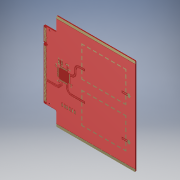
# Autodesk Inventor part: RCS_PCB
Saved by Autodesk Inventor 2018 (Build 220112000, 112)
## iProperties
Created: 2018-01-15
Part Number: RCS_PCB
Material: Epoxy Resin
Document SubType Name: Modeling
Designer: Bradley
Density: 1.14 g/cm^3
Appearance: Red
Author: Bradley
Revision Number: 3
Autodesk Inventor part; units mm, degrees
(part 1 of 4)
ref_plane "YZ Plane" through (0, 0, 0) normal (1, 0, 0) x (0, 1, 0)
ref_plane "XZ Plane" through (0, 0, 0) normal (0, 1, 0) x (-1, 0, 0)
ref_plane "XY Plane" through (0, 0, 0) normal (0, 0, 1) x (1, 0, 0)
sketch "Sketch1" plane through (0, 0, 0) normal (0, 0, 1) x (1, 0, 0)
  line L0 (0, 33.8) -> (12.5, 33.8)
  line L1 (12.5, 33.8) -> (12.5, 47.9)
  line L2 (12.5, 47.9) -> (91.4, 47.9)
  line L3 (91.4, 47.9) -> (91.4, -47.9)
  line L4 (91.4, -47.9) -> (12.5, -47.9)
  line L5 (12.5, -47.9) -> (12.5, -33.8)
  line L6 (12.5, -33.8) -> (0, -33.8)
  line L7 (0, -33.8) -> (0, 33.8)
  line L8 (-4.5, 48) -> (91.5, 48) construction
  line L9 (91.5, 48) -> (91.5, -48) construction
  line L10 (91.5, -48) -> (-4.5, -48) construction
  line L11 (-4.5, -48) -> (-4.5, 48) construction
  line L12 (-4.4, 47.9) -> (-3.4, 47.9) construction
  line L13 (-3.4, 47.9) -> (-3.4, -47.9) construction
  line L14 (-3.4, -47.9) -> (-4.4, -47.9) construction
  line L15 (-4.4, -47.9) -> (-4.4, 47.9) construction
  point P0 (0, 0)
  point P1 (0, 0)
  point P2 (-4.5, 0)
  dimension "d0" = 67.6
  dimension "d1" = 95.8
  dimension "d2" = 91.4
  dimension "d3" = 12.5
  dimension "d20" = 96
  dimension "d21" = 96
  dimension "d22" = 0.1
  dimension "d23" = 0.1
  dimension "d24" = 1
  dimension "d25" = 0.1
  dimension "d26" = 3.4
  constraints: 32 end point, 8 perpendicular, 4 parallel, 3 collinear, 3 horizontal, 2 midpoint, 2 point on line, 1 coincident, 1 horizontal alignment
  measures "d0" distance of L6.end L0.start
  measures "d1" distance of L2.end L3.end
  measures "d2" distance between parallel lines of L7 L3
  measures "d3" distance of L0.start L0.end
  measures "d20" distance of L8.start L8.end
  measures "d21" distance of L10.end L8.start
  measures "d22" distance between parallel lines of L2 L8
  measures "d23" distance between parallel lines of L9 L3
  measures "d24" distance between parallel lines of L15 L13
  measures "d25" distance between parallel lines of L15 L11
  measures "d26" distance between parallel lines of L7 L13
extrude "Extrusion1" add sketch "Sketch1" along normal mid plane 1
sketch "Sketch2" plane through (0, 0, 0.5) normal (0, 0, 1) x (1, 0, 0)
  line L0 (12.5, 33.8) -> (0, 33.8)
  line L1 (0, 33.8) -> (0, -33.8)
  line L2 (0, -33.8) -> (12.5, -33.8)
  line L3 (12.5, -33.8) -> (12.5, -47.9)
  line L4 (12.5, -47.9) -> (91.4, -47.9)
  line L5 (91.4, -47.9) -> (91.4, 47.9)
  line L6 (91.4, 47.9) -> (12.5, 47.9)
  line L7 (12.5, 47.9) -> (12.5, 33.8)
  line L8 (91.4, -47.9) -> (91.4, 47.9)
  line L9 (12.5, 47.9) -> (91.4, 47.9)
  line L10 (91.4, 47.9) -> (91.4, 45.4)
  line L11 (91.4, 45.4) -> (12.5, 45.4)
  line L12 (12.5, 45.4) -> (12.5, 47.9)
  line L13 (91.4, -47.9) -> (12.5, -47.9)
  line L14 (12.5, -47.9) -> (12.5, -45.4)
  line L15 (12.5, -45.4) -> (91.4, -45.4)
  line L16 (91.4, -45.4) -> (91.4, -47.9)
  point P0 (0, 0)
  dimension "d6" = 2.5
  dimension "d27" = 90.8
  constraints: 16 end point, 4 parallel, 2 horizontal, 2 perpendicular, 2 point on line, 1 collinear
  measures "d6" distance between parallel lines of L4 L15
  measures "d27" distance between parallel lines of L15 L11
extrude "Extrusion2" add sketch "Sketch2" along normal blind 0.01 contours L7 L6 L5 L11 | L5 L4 L3 L15
mirror "Mirror1" about plane through (0, 0, 0) normal (0, 0, 1) of "Extrusion2"
sketch "Sketch3" plane through (0, 0, 0.5) normal (0, 0, 1) x (1, 0, 0)
  circle A0 centre (6, 31.8) radius 0.9
  circle A1 centre (6, -31.8) radius 0.9
  point P0 (0, 0)
  dimension "d9" = 1.8
  dimension "d10" = 6
  dimension "d11" = 31.8
  dimension "d12" = 31.8
  constraints: 2 centre point, 1 equal radius, 1 vertical alignment
  measures "d9" diameter of A0
  measures "d10" horizontal distance of point (0, 0) A0.centre
  measures "d11" vertical distance of point (0, 0) A0.centre
  measures "d12" vertical distance of A1.centre point (0, 0)
extrude "Extrusion3" cut sketch "Sketch3" against normal through all
sketch "Sketch4" plane through (0, 0, 0.5) normal (0, 0, 1) x (1, 0, 0)
  circle A0 centre (6, 31.8) radius 0.9
  circle A1 centre (6, -31.8) radius 0.9
  line L0 (12.5, -45.4) -> (91.4, -45.4)
  line L1 (91.4, -45.4) -> (91.4, 45.4)
  line L2 (91.4, 45.4) -> (12.5, 45.4)
  line L3 (12.5, 45.4) -> (12.5, 33.8)
  line L4 (12.5, 33.8) -> (0, 33.8)
  line L5 (0, 33.8) -> (0, -33.8)
  line L6 (0, -33.8) -> (12.5, -33.8)
  line L7 (12.5, -33.8) -> (12.5, -45.4)
  line L8 (0, 18.95) -> (3.5, 18.95)
  arc A2 (3.5, 17.95) -> (3.5, 18.95) centre (3.5, 18.45) ccw
  line L9 (3.5, 17.95) -> (0, 17.95)
  point P0 (0, 0)
  dimension "d15" = 17.95
  dimension "d16" = 3.5
  dimension "d17" = 1
  constraints: 4 end point, 2 point on circle, 2 point on line, 2 tangent, 1 centre point, 1 horizontal, 1 perpendicular
  measures "d15" distance from line of point (0, 0) L9
  measures "d16" distance from line of A2.centre L5
  measures "d17" distance between parallel lines of L9 L8
extrude "Extrusion4" cut sketch "Sketch4" against normal through all contours L5 L8 A2 L9
sketch "Sketch5" plane through (0, 0, 0.5) normal (0, 0, 1) x (1, 0, 0)
  line L0 (37.6, 36.65) -> (82.4, 36.65)
  line L1 (82.4, 36.65) -> (82.4, 5.35)
  line L2 (82.4, 5.35) -> (37.6, 5.35)
  line L3 (37.6, 5.35) -> (37.6, 36.65)
  line L4 (81.4, 35.65) -> (38.6, 35.65)
  line L5 (38.6, 35.65) -> (38.6, 6.35)
  line L6 (38.6, 6.35) -> (81.4, 6.35)
  line L7 (81.4, 6.35) -> (81.4, 35.65)
  line L8 (37.6, 7.9) -> (38.6, 7.9)
  line L9 (37.6, 10.1) -> (38.6, 10.1)
  line L10 (37.6, 13.9) -> (38.6, 13.9)
  line L11 (37.6, 16.1) -> (38.6, 16.1)
  line L12 (37.6, 19.9) -> (38.6, 19.9)
  line L13 (37.6, 22.1) -> (38.6, 22.1)
  line L14 (37.6, 25.9) -> (38.6, 25.9)
  line L15 (37.6, 28.1) -> (38.6, 28.1)
  line L16 (37.6, 31.9) -> (38.6, 31.9)
  line L17 (37.6, 34.1) -> (38.6, 34.1)
  line L18 (81.4, 34.1) -> (82.4, 34.1)
  line L19 (81.4, 31.9) -> (82.4, 31.9)
  line L20 (81.4, 28.1) -> (82.4, 28.1)
  line L21 (81.4, 25.9) -> (82.4, 25.9)
  line L22 (81.4, 22.1) -> (82.4, 22.1)
  line L23 (81.4, 19.9) -> (82.4, 19.9)
  line L24 (81.4, 16.1) -> (82.4, 16.1)
  line L25 (81.4, 13.9) -> (82.4, 13.9)
  line L26 (81.4, 10.1) -> (82.4, 10.1)
  line L27 (81.4, 7.9) -> (82.4, 7.9)
  line L28 (40.9, 6.35) -> (40.9, 5.35)
  line L29 (43.1, 6.35) -> (43.1, 5.35)
  line L30 (46.9, 6.35) -> (46.9, 5.35)
  line L31 (49.1, 6.35) -> (49.1, 5.35)
  line L32 (52.9, 6.35) -> (52.9, 5.35)
  line L33 (55.1, 6.35) -> (55.1, 5.35)
  line L34 (58.9, 6.35) -> (58.9, 5.35)
  line L35 (61.1, 6.35) -> (61.1, 5.35)
  line L36 (64.9, 6.35) -> (64.9, 5.35)
  line L37 (67.1, 6.35) -> (67.1, 5.35)
  line L38 (67.1, 36.65) -> (67.1, 35.65)
  line L39 (64.9, 36.65) -> (64.9, 35.65)
  line L40 (61.1, 36.65) -> (61.1, 35.65)
  line L41 (58.9, 36.65) -> (58.9, 35.65)
  line L42 (55.1, 36.65) -> (55.1, 35.65)
  line L43 (52.9, 36.65) -> (52.9, 35.65)
  line L44 (49.1, 36.65) -> (49.1, 35.65)
  line L45 (46.9, 36.65) -> (46.9, 35.65)
  line L46 (43.1, 36.65) -> (43.1, 35.65)
  line L47 (40.9, 35.65) -> (40.9, 36.65)
  line L48 (83.9, 13.25) -> (86.1, 13.25)
  line L49 (86.1, 13.25) -> (86.1, 16.75)
  line L50 (86.1, 16.75) -> (83.9, 16.75)
  line L51 (83.9, 16.75) -> (83.9, 13.25)
  line L52 (83.9, 14.6) -> (83.4, 14.6)
  line L53 (83.4, 14.6) -> (83.4, 15.4)
  line L54 (83.4, 15.4) -> (83.9, 15.4)
  line L55 (83.9, 15.4) -> (83.9, 14.6)
  line L56 (86.1, 14.6) -> (86.6, 14.6)
  line L57 (86.6, 14.6) -> (86.6, 15.4)
  line L58 (86.6, 15.4) -> (86.1, 15.4)
  line L59 (86.1, 15.4) -> (86.1, 14.6)
  line L60 (70.9, 6.35) -> (70.9, 5.35)
  line L61 (73.1, 6.35) -> (73.1, 5.35)
  line L62 (76.9, 6.35) -> (76.9, 5.35)
  line L63 (79.1, 6.35) -> (79.1, 5.35)
  line L64 (79.1, 35.65) -> (79.1, 36.65)
  line L65 (76.9, 36.65) -> (76.9, 35.65)
  line L66 (73.1, 35.65) -> (73.1, 36.65)
  line L67 (70.9, 36.65) -> (70.9, 35.65)
  point P0 (0, 0)
  point P1 (38.6, 21)
  point P2 (60, 35.65)
  point P3 (83.9, 15)
  point P4 (85, 16.75)
  dimension "d30" = 1
  dimension "d28" = 31.3
  dimension "d29" = 44.8
  dimension "d31" = 60
  dimension "d32" = 21
  dimension "d33" = 2.55
  dimension "d34" = 4.75
  dimension "d35" = 8.55
  dimension "d36" = 10.75
  dimension "d37" = 14.55
  dimension "d38" = 16.75
  dimension "d39" = 20.55
  dimension "d40" = 22.75
  dimension "d41" = 26.55
  dimension "d42" = 28.75
  dimension "d43" = 3.3
  dimension "d44" = 5.5
  dimension "d45" = 9.3
  dimension "d46" = 11.5
  dimension "d47" = 15.3
  dimension "d48" = 17.5
  dimension "d49" = 21.3
  dimension "d50" = 23.5
  dimension "d51" = 27.3
  dimension "d52" = 29.5
  dimension "d55" = 2.2
  dimension "d56" = 3.5
  dimension "d57" = 0.5
  dimension "d58" = 0.8
  dimension "d59" = 15
  dimension "d60" = 85
  dimension "d64" = 33.3
  dimension "d65" = 35.5
  dimension "d66" = 39.3
  dimension "d67" = 41.5
  constraints: 120 end point, 42 point on line, 17 horizontal, 14 vertical, 7 collinear, 6 parallel, 3 midpoint, 3 perpendicular, 122 other
  measures "d28" distance of point (37.6, 5.35) point (37.6, 36.65)
  measures "d29" distance of point (82.4, 5.35) point (37.6, 5.35)
  measures "d31" horizontal distance of point (0, 0) point (60, 35.65)
  measures "d32" vertical distance of point (0, 0) point (38.6, 21)
  measures "d55" distance of L49.end L50.end
  measures "d56" distance of L48.end L49.end
  measures "d57" distance of L53.end L54.end
  measures "d58" distance of L52.end L53.end
  measures "d59" vertical distance of point (83.9, 15) point (0, 0)
  measures "d60" horizontal distance of point (0, 0) point (85, 16.75)
extrude "Extrusion5" add sketch "Sketch5" along normal blind 0.035 contours L0 L47 L4 L5 L17 L3 | L0 L45 L4 L46 | L16 L5 L15 L3 | L0 L43 L4 L44 | L14 L5 L13 L3 | L0 L41 L4 L42 | L12 L5 L11 L3 | L0 L39 L4 L40 | L10 L5 L9 L3 | L0 L67 L4 L38 | L8 L5 L6 L28 L2 L3 | L0 L65 L4 L66 | L29 L6 L30 L2 | L0 L1 L18 L7 L4 L64 | L31 L6 L32 L2 | L1 L20 L7 L19 | L33 L6 L34 L2 | L1 L22 L7 L21 | L35 L6 L36 L2 | L1 L24 L7 L23 | L37 L6 L60 L2 | L1 L26 L7 L25 | L61 L6 L62 L2 | L1 L2 L63 L6 L7 L27 | L51 L50 L49 L48 | L52 L53 L54 L51 | L49 L58 L57 L56
pattern_linear "Rectangular Pattern1" count 2 spacing 40 along (0, -1, 0) of "Extrusion5"
sketch "Sketch6" plane through (0, 0, 0.5) normal (0, 0, 1) x (1, 0, 0)
  line L0 (79.1, -4.35) -> (79.1, -3.35)
  line L1 (79.1, -3.35) -> (82.4, -3.35)
  line L2 (82.4, -3.35) -> (82.4, -5.9)
  line L3 (82.4, -5.9) -> (81.4, -5.9)
  line L4 (81.4, -5.9) -> (81.4, -4.35)
  line L5 (81.4, -4.35) -> (79.1, -4.35)
  line L6 (37.6, -34.65) -> (37.6, -32.1)
  line L7 (37.6, -32.1) -> (38.6, -32.1)
  line L8 (38.6, -32.1) -> (38.6, -33.65)
  line L9 (38.6, -33.65) -> (40.9, -33.65)
  line L10 (40.9, -33.65) -> (40.9, -34.65)
  line L11 (40.9, -34.65) -> (37.6, -34.65)
  line L12 (70.9, -3.35) -> (70.9, -4.35)
  line L13 (70.9, -4.35) -> (67.1, -4.35)
  line L14 (67.1, -4.35) -> (67.1, -3.35)
  line L15 (67.1, -3.35) -> (70.9, -3.35)
  line L16 (73.1, -33.65) -> (76.9, -33.65)
  line L17 (76.9, -33.65) -> (76.9, -34.65)
  line L18 (76.9, -34.65) -> (73.1, -34.65)
  line L19 (73.1, -34.65) -> (73.1, -33.65)
  line L20 (81.4, -20.1) -> (82.4, -20.1)
  line L21 (82.4, -20.1) -> (82.4, -23.9)
  line L22 (82.4, -23.9) -> (81.4, -23.9)
  line L23 (81.4, -23.9) -> (81.4, -20.1)
  line L24 (46.9, -3.35) -> (46.9, -4.35)
  line L25 (46.9, -4.35) -> (43.1, -4.35)
  line L26 (43.1, -4.35) -> (43.1, -3.35)
  line L27 (43.1, -3.35) -> (46.9, -3.35)
  line L28 (58.9, -3.35) -> (58.9, -4.35)
  line L29 (58.9, -4.35) -> (55.1, -4.35)
  line L30 (55.1, -4.35) -> (55.1, -3.35)
  line L31 (55.1, -3.35) -> (58.9, -3.35)
  line L32 (61.1, -33.65) -> (64.9, -33.65)
  line L33 (64.9, -33.65) -> (64.9, -34.65)
  line L34 (64.9, -34.65) -> (61.1, -34.65)
  line L35 (61.1, -34.65) -> (61.1, -33.65)
  line L36 (49.1, -33.65) -> (52.9, -33.65)
  line L37 (52.9, -33.65) -> (52.9, -34.65)
  line L38 (52.9, -34.65) -> (49.1, -34.65)
  line L39 (49.1, -34.65) -> (49.1, -33.65)
  line L40 (81.4, -26.1) -> (82.4, -26.1)
  line L41 (82.4, -26.1) -> (82.4, -29.9)
  line L42 (82.4, -29.9) -> (81.4, -29.9)
  line L43 (81.4, -29.9) -> (81.4, -26.1)
  line L44 (81.4, -8.1) -> (82.4, -8.1)
  line L45 (82.4, -8.1) -> (82.4, -11.9)
  line L46 (82.4, -11.9) -> (81.4, -11.9)
  line L47 (81.4, -11.9) -> (81.4, -8.1)
  line L48 (37.6, -17.9) -> (37.6, -14.1)
  line L49 (37.6, -14.1) -> (38.6, -14.1)
  line L50 (38.6, -14.1) -> (38.6, -17.9)
  line L51 (38.6, -17.9) -> (37.6, -17.9)
  line L52 (86.1, -25.4) -> (86.1, -26.75)
  line L53 (86.1, -26.75) -> (83.9, -26.75)
  line L54 (83.9, -26.75) -> (83.9, -25.4)
  line L55 (83.9, -25.4) -> (83.4, -25.4)
  line L56 (83.4, -25.4) -> (83.4, -24.6)
  line L57 (83.4, -24.6) -> (83.9, -24.6)
  line L58 (83.9, -24.6) -> (83.9, -23.25)
  line L59 (83.9, -23.25) -> (86.1, -23.25)
  line L60 (86.1, -23.25) -> (86.1, -24.6)
  line L61 (86.1, -24.6) -> (86.6, -24.6)
  line L62 (86.6, -24.6) -> (86.6, -25.4)
  line L63 (86.6, -25.4) -> (86.1, -25.4)
  line L64 (37.6, -29.9) -> (37.6, -26.1)
  line L65 (37.6, -26.1) -> (38.6, -26.1)
  line L66 (38.6, -26.1) -> (38.6, -29.9)
  line L67 (38.6, -29.9) -> (37.6, -29.9)
  line L68 (37.6, -11.9) -> (37.6, -8.1)
  line L69 (37.6, -8.1) -> (38.6, -8.1)
  line L70 (38.6, -8.1) -> (38.6, -11.9)
  line L71 (38.6, -11.9) -> (37.6, -11.9)
  line L72 (81.4, -14.1) -> (82.4, -14.1)
  line L73 (82.4, -14.1) -> (82.4, -17.9)
  line L74 (82.4, -17.9) -> (81.4, -17.9)
  line L75 (81.4, -17.9) -> (81.4, -14.1)
  line L76 (43.1, -33.65) -> (46.9, -33.65)
  line L77 (46.9, -33.65) -> (46.9, -34.65)
  line L78 (46.9, -34.65) -> (43.1, -34.65)
  line L79 (43.1, -34.65) -> (43.1, -33.65)
  line L80 (55.1, -33.65) -> (58.9, -33.65)
  line L81 (58.9, -33.65) -> (58.9, -34.65)
  line L82 (58.9, -34.65) -> (55.1, -34.65)
  line L83 (55.1, -34.65) -> (55.1, -33.65)
  line L84 (64.9, -3.35) -> (64.9, -4.35)
  line L85 (64.9, -4.35) -> (61.1, -4.35)
  line L86 (61.1, -4.35) -> (61.1, -3.35)
  line L87 (61.1, -3.35) -> (64.9, -3.35)
  line L88 (52.9, -3.35) -> (52.9, -4.35)
  line L89 (52.9, -4.35) -> (49.1, -4.35)
  line L90 (49.1, -4.35) -> (49.1, -3.35)
  line L91 (49.1, -3.35) -> (52.9, -3.35)
  line L92 (37.6, -23.9) -> (37.6, -20.1)
  line L93 (37.6, -20.1) -> (38.6, -20.1)
  line L94 (38.6, -20.1) -> (38.6, -23.9)
  line L95 (38.6, -23.9) -> (37.6, -23.9)
  line L96 (70.9, -33.65) -> (70.9, -34.65)
  line L97 (70.9, -34.65) -> (67.1, -34.65)
  line L98 (67.1, -34.65) -> (67.1, -33.65)
  line L99 (67.1, -33.65) -> (70.9, -33.65)
  line L100 (76.9, -3.35) -> (76.9, -4.35)
  line L101 (76.9, -4.35) -> (73.1, -4.35)
  line L102 (73.1, -4.35) -> (73.1, -3.35)
  line L103 (73.1, -3.35) -> (76.9, -3.35)
  line L104 (37.6, -3.35) -> (40.9, -3.35)
  line L105 (40.9, -3.35) -> (40.9, -4.35)
  line L106 (40.9, -4.35) -> (38.6, -4.35)
  line L107 (38.6, -4.35) -> (38.6, -5.9)
  line L108 (38.6, -5.9) -> (37.6, -5.9)
  line L109 (37.6, -5.9) -> (37.6, -3.35)
  line L110 (79.1, -33.65) -> (81.4, -33.65)
  line L111 (81.4, -33.65) -> (81.4, -32.1)
  line L112 (81.4, -32.1) -> (82.4, -32.1)
  line L113 (82.4, -32.1) -> (82.4, -34.65)
  line L114 (82.4, -34.65) -> (79.1, -34.65)
  line L115 (79.1, -34.65) -> (79.1, -33.65)
  line L116 (79.1, 35.65) -> (79.1, 36.65)
  line L117 (79.1, 36.65) -> (82.4, 36.65)
  line L118 (82.4, 36.65) -> (82.4, 34.1)
  line L119 (82.4, 34.1) -> (81.4, 34.1)
  line L120 (81.4, 34.1) -> (81.4, 35.65)
  line L121 (81.4, 35.65) -> (79.1, 35.65)
  line L122 (37.6, 5.35) -> (37.6, 7.9)
  line L123 (37.6, 7.9) -> (38.6, 7.9)
  line L124 (38.6, 7.9) -> (38.6, 6.35)
  line L125 (38.6, 6.35) -> (40.9, 6.35)
  line L126 (40.9, 6.35) -> (40.9, 5.35)
  line L127 (40.9, 5.35) -> (37.6, 5.35)
  line L128 (70.9, 36.65) -> (70.9, 35.65)
  line L129 (70.9, 35.65) -> (67.1, 35.65)
  line L130 (67.1, 35.65) -> (67.1, 36.65)
  line L131 (67.1, 36.65) -> (70.9, 36.65)
  line L132 (73.1, 6.35) -> (76.9, 6.35)
  line L133 (76.9, 6.35) -> (76.9, 5.35)
  line L134 (76.9, 5.35) -> (73.1, 5.35)
  line L135 (73.1, 5.35) -> (73.1, 6.35)
  line L136 (81.4, 19.9) -> (82.4, 19.9)
  line L137 (82.4, 19.9) -> (82.4, 16.1)
  line L138 (82.4, 16.1) -> (81.4, 16.1)
  line L139 (81.4, 16.1) -> (81.4, 19.9)
  line L140 (46.9, 36.65) -> (46.9, 35.65)
  line L141 (46.9, 35.65) -> (43.1, 35.65)
  line L142 (43.1, 35.65) -> (43.1, 36.65)
  line L143 (43.1, 36.65) -> (46.9, 36.65)
  line L144 (58.9, 36.65) -> (58.9, 35.65)
  line L145 (58.9, 35.65) -> (55.1, 35.65)
  line L146 (55.1, 35.65) -> (55.1, 36.65)
  line L147 (55.1, 36.65) -> (58.9, 36.65)
  line L148 (61.1, 6.35) -> (64.9, 6.35)
  line L149 (64.9, 6.35) -> (64.9, 5.35)
  line L150 (64.9, 5.35) -> (61.1, 5.35)
  line L151 (61.1, 5.35) -> (61.1, 6.35)
  line L152 (49.1, 6.35) -> (52.9, 6.35)
  line L153 (52.9, 6.35) -> (52.9, 5.35)
  line L154 (52.9, 5.35) -> (49.1, 5.35)
  line L155 (49.1, 5.35) -> (49.1, 6.35)
  line L156 (81.4, 13.9) -> (82.4, 13.9)
  line L157 (82.4, 13.9) -> (82.4, 10.1)
  line L158 (82.4, 10.1) -> (81.4, 10.1)
  line L159 (81.4, 10.1) -> (81.4, 13.9)
  line L160 (81.4, 31.9) -> (82.4, 31.9)
  line L161 (82.4, 31.9) -> (82.4, 28.1)
  line L162 (82.4, 28.1) -> (81.4, 28.1)
  line L163 (81.4, 28.1) -> (81.4, 31.9)
  line L164 (37.6, 22.1) -> (37.6, 25.9)
  line L165 (37.6, 25.9) -> (38.6, 25.9)
  line L166 (38.6, 25.9) -> (38.6, 22.1)
  line L167 (38.6, 22.1) -> (37.6, 22.1)
  line L168 (86.1, 14.6) -> (86.1, 13.25)
  line L169 (86.1, 13.25) -> (83.9, 13.25)
  line L170 (83.9, 13.25) -> (83.9, 14.6)
  line L171 (83.9, 14.6) -> (83.4, 14.6)
  line L172 (83.4, 14.6) -> (83.4, 15.4)
  line L173 (83.4, 15.4) -> (83.9, 15.4)
  line L174 (83.9, 15.4) -> (83.9, 16.75)
  line L175 (83.9, 16.75) -> (86.1, 16.75)
  line L176 (86.1, 16.75) -> (86.1, 15.4)
  line L177 (86.1, 15.4) -> (86.6, 15.4)
  line L178 (86.6, 15.4) -> (86.6, 14.6)
  line L179 (86.6, 14.6) -> (86.1, 14.6)
  line L180 (37.6, 10.1) -> (37.6, 13.9)
  line L181 (37.6, 13.9) -> (38.6, 13.9)
  line L182 (38.6, 13.9) -> (38.6, 10.1)
  line L183 (38.6, 10.1) -> (37.6, 10.1)
  line L184 (37.6, 28.1) -> (37.6, 31.9)
  line L185 (37.6, 31.9) -> (38.6, 31.9)
  line L186 (38.6, 31.9) -> (38.6, 28.1)
  line L187 (38.6, 28.1) -> (37.6, 28.1)
  line L188 (81.4, 25.9) -> (82.4, 25.9)
  line L189 (82.4, 25.9) -> (82.4, 22.1)
  line L190 (82.4, 22.1) -> (81.4, 22.1)
  line L191 (81.4, 22.1) -> (81.4, 25.9)
  line L192 (43.1, 6.35) -> (46.9, 6.35)
  line L193 (46.9, 6.35) -> (46.9, 5.35)
  line L194 (46.9, 5.35) -> (43.1, 5.35)
  line L195 (43.1, 5.35) -> (43.1, 6.35)
  line L196 (55.1, 6.35) -> (58.9, 6.35)
  line L197 (58.9, 6.35) -> (58.9, 5.35)
  line L198 (58.9, 5.35) -> (55.1, 5.35)
  line L199 (55.1, 5.35) -> (55.1, 6.35)
  line L200 (64.9, 36.65) -> (64.9, 35.65)
  line L201 (64.9, 35.65) -> (61.1, 35.65)
  line L202 (61.1, 35.65) -> (61.1, 36.65)
  line L203 (61.1, 36.65) -> (64.9, 36.65)
  line L204 (52.9, 36.65) -> (52.9, 35.65)
  line L205 (52.9, 35.65) -> (49.1, 35.65)
  line L206 (49.1, 35.65) -> (49.1, 36.65)
  line L207 (49.1, 36.65) -> (52.9, 36.65)
  line L208 (37.6, 16.1) -> (37.6, 19.9)
  line L209 (37.6, 19.9) -> (38.6, 19.9)
  line L210 (38.6, 19.9) -> (38.6, 16.1)
  line L211 (38.6, 16.1) -> (37.6, 16.1)
  line L212 (70.9, 6.35) -> (70.9, 5.35)
  line L213 (70.9, 5.35) -> (67.1, 5.35)
  line L214 (67.1, 5.35) -> (67.1, 6.35)
  line L215 (67.1, 6.35) -> (70.9, 6.35)
  line L216 (76.9, 36.65) -> (76.9, 35.65)
  line L217 (76.9, 35.65) -> (73.1, 35.65)
  line L218 (73.1, 35.65) -> (73.1, 36.65)
  line L219 (73.1, 36.65) -> (76.9, 36.65)
  line L220 (37.6, 36.65) -> (40.9, 36.65)
  line L221 (40.9, 36.65) -> (40.9, 35.65)
  line L222 (40.9, 35.65) -> (38.6, 35.65)
  line L223 (38.6, 35.65) -> (38.6, 34.1)
  line L224 (38.6, 34.1) -> (37.6, 34.1)
  line L225 (37.6, 34.1) -> (37.6, 36.65)
  line L226 (79.1, 6.35) -> (81.4, 6.35)
  line L227 (81.4, 6.35) -> (81.4, 7.9)
  line L228 (81.4, 7.9) -> (82.4, 7.9)
  line L229 (82.4, 7.9) -> (82.4, 5.35)
  line L230 (82.4, 5.35) -> (79.1, 5.35)
  line L231 (79.1, 5.35) -> (79.1, 6.35)
  line L232 (0, 18.95) -> (3.5, 18.95)
  arc A0 (3.5, 17.95) -> (3.5, 18.95) centre (3.5, 18.45) ccw
  line L233 (3.5, 17.95) -> (0, 17.95)
  line L234 (0, 17.95) -> (0, -33.8)
  line L235 (0, -33.8) -> (12.5, -33.8)
  line L236 (12.5, -33.8) -> (12.5, -45.4)
  line L237 (12.5, -45.4) -> (91.4, -45.4)
  line L238 (91.4, -45.4) -> (91.4, 45.4)
  line L239 (91.4, 45.4) -> (12.5, 45.4)
  line L240 (12.5, 45.4) -> (12.5, 33.8)
  line L241 (12.5, 33.8) -> (0, 33.8)
  line L242 (0, 33.8) -> (0, 18.95)
  circle A1 centre (6, -31.8) radius 0.9
  circle A2 centre (6, 31.8) radius 0.9
  line L243 (18, -25) -> (19, -25)
  line L244 (19, -25) -> (19, -27.5)
  line L245 (19, -27.5) -> (18, -27.5)
  line L246 (18, -27.5) -> (18, -25)
  line L247 (21.54, -27.5) -> (20.54, -27.5)
  line L248 (21.54, -25) -> (21.54, -27.5)
  line L249 (20.54, -25) -> (21.54, -25)
  line L250 (20.54, -27.5) -> (20.54, -25)
  line L251 (24.08, -27.5) -> (23.08, -27.5)
  line L252 (24.08, -25) -> (24.08, -27.5)
  line L253 (23.08, -25) -> (24.08, -25)
  line L254 (23.08, -27.5) -> (23.08, -25)
  line L255 (26.62, -27.5) -> (25.62, -27.5)
  line L256 (26.62, -25) -> (26.62, -27.5)
  line L257 (25.62, -25) -> (26.62, -25)
  line L258 (25.62, -27.5) -> (25.62, -25)
  line L259 (29.16, -27.5) -> (28.16, -27.5)
  line L260 (29.16, -25) -> (29.16, -27.5)
  line L261 (28.16, -25) -> (29.16, -25)
  line L262 (28.16, -27.5) -> (28.16, -25)
  line L263 (31.7, -27.5) -> (30.7, -27.5)
  line L264 (31.7, -25) -> (31.7, -27.5)
  line L265 (30.7, -25) -> (31.7, -25)
  line L266 (30.7, -27.5) -> (30.7, -25)
  line L267 (16.1, 6.35) -> (16.4, 6.35)
  line L268 (16.4, 6.35) -> (16.4, 5.15)
  line L269 (16.4, 5.15) -> (16.1, 5.15)
  line L270 (16.1, 5.15) -> (16.1, 6.35)
  line L271 (16.1, -5.15) -> (16.4, -5.15)
  line L272 (16.4, -5.15) -> (16.4, -6.35)
  line L273 (16.4, -6.35) -> (16.1, -6.35)
  line L274 (16.1, -6.35) -> (16.1, -5.15)
  line L275 (16.6, 6.35) -> (16.9, 6.35)
  line L276 (16.6, 5.15) -> (16.6, 6.35)
  line L277 (16.9, 6.35) -> (16.9, 5.15)
  line L278 (16.6, -5.15) -> (16.9, -5.15)
  line L279 (16.6, -6.35) -> (16.6, -5.15)
  line L280 (16.9, -6.35) -> (16.6, -6.35)
  line L281 (16.9, -5.15) -> (16.9, -6.35)
  line L282 (16.9, 5.15) -> (16.6, 5.15)
  line L283 (17.1, 6.35) -> (17.4, 6.35)
  line L284 (17.1, 5.15) -> (17.1, 6.35)
  line L285 (17.4, 6.35) -> (17.4, 5.15)
  line L286 (17.1, -5.15) -> (17.4, -5.15)
  line L287 (17.1, -6.35) -> (17.1, -5.15)
  line L288 (17.4, -6.35) -> (17.1, -6.35)
  line L289 (17.4, -5.15) -> (17.4, -6.35)
  line L290 (17.4, 5.15) -> (17.1, 5.15)
  line L291 (17.6, 6.35) -> (17.9, 6.35)
  line L292 (17.6, 5.15) -> (17.6, 6.35)
  line L293 (17.9, 6.35) -> (17.9, 5.15)
  line L294 (17.6, -5.15) -> (17.9, -5.15)
  line L295 (17.6, -6.35) -> (17.6, -5.15)
  line L296 (17.9, -6.35) -> (17.6, -6.35)
  line L297 (17.9, -5.15) -> (17.9, -6.35)
  line L298 (17.9, 5.15) -> (17.6, 5.15)
  line L299 (18.1, 6.35) -> (18.4, 6.35)
  line L300 (18.1, 5.15) -> (18.1, 6.35)
  line L301 (18.4, 6.35) -> (18.4, 5.15)
  line L302 (18.1, -5.15) -> (18.4, -5.15)
  line L303 (18.1, -6.35) -> (18.1, -5.15)
  line L304 (18.4, -6.35) -> (18.1, -6.35)
  line L305 (18.4, -5.15) -> (18.4, -6.35)
  line L306 (18.4, 5.15) -> (18.1, 5.15)
  line L307 (18.6, 6.35) -> (18.9, 6.35)
  line L308 (18.6, 5.15) -> (18.6, 6.35)
  line L309 (18.9, 6.35) -> (18.9, 5.15)
  line L310 (18.6, -5.15) -> (18.9, -5.15)
  line L311 (18.6, -6.35) -> (18.6, -5.15)
  line L312 (18.9, -6.35) -> (18.6, -6.35)
  line L313 (18.9, -5.15) -> (18.9, -6.35)
  line L314 (18.9, 5.15) -> (18.6, 5.15)
  line L315 (19.1, 6.35) -> (19.4, 6.35)
  line L316 (19.1, 5.15) -> (19.1, 6.35)
  line L317 (19.4, 6.35) -> (19.4, 5.15)
  line L318 (19.1, -5.15) -> (19.4, -5.15)
  line L319 (19.1, -6.35) -> (19.1, -5.15)
  line L320 (19.4, -6.35) -> (19.1, -6.35)
  line L321 (19.4, -5.15) -> (19.4, -6.35)
  line L322 (19.4, 5.15) -> (19.1, 5.15)
  line L323 (19.6, 6.35) -> (19.9, 6.35)
  line L324 (19.6, 5.15) -> (19.6, 6.35)
  line L325 (19.9, 6.35) -> (19.9, 5.15)
  line L326 (19.6, -5.15) -> (19.9, -5.15)
  line L327 (19.6, -6.35) -> (19.6, -5.15)
  line L328 (19.9, -6.35) -> (19.6, -6.35)
  line L329 (19.9, -5.15) -> (19.9, -6.35)
  line L330 (19.9, 5.15) -> (19.6, 5.15)
  line L331 (20.1, 6.35) -> (20.4, 6.35)
  line L332 (20.1, 5.15) -> (20.1, 6.35)
  line L333 (20.4, 6.35) -> (20.4, 5.15)
  line L334 (20.1, -5.15) -> (20.4, -5.15)
  line L335 (20.1, -6.35) -> (20.1, -5.15)
  line L336 (20.4, -6.35) -> (20.1, -6.35)
  line L337 (20.4, -5.15) -> (20.4, -6.35)
  line L338 (20.4, 5.15) -> (20.1, 5.15)
  line L339 (20.6, 6.35) -> (20.9, 6.35)
  line L340 (20.6, 5.15) -> (20.6, 6.35)
  line L341 (20.9, 6.35) -> (20.9, 5.15)
  line L342 (20.6, -5.15) -> (20.9, -5.15)
  line L343 (20.6, -6.35) -> (20.6, -5.15)
  line L344 (20.9, -6.35) -> (20.6, -6.35)
  line L345 (20.9, -5.15) -> (20.9, -6.35)
  line L346 (20.9, 5.15) -> (20.6, 5.15)
  line L347 (21.1, 6.35) -> (21.4, 6.35)
  line L348 (21.1, 5.15) -> (21.1, 6.35)
  line L349 (21.4, 6.35) -> (21.4, 5.15)
  line L350 (21.1, -5.15) -> (21.4, -5.15)
  line L351 (21.1, -6.35) -> (21.1, -5.15)
  line L352 (21.4, -6.35) -> (21.1, -6.35)
  line L353 (21.4, -5.15) -> (21.4, -6.35)
  line L354 (21.4, 5.15) -> (21.1, 5.15)
  line L355 (21.6, 6.35) -> (21.9, 6.35)
  line L356 (21.6, 5.15) -> (21.6, 6.35)
  line L357 (21.9, 6.35) -> (21.9, 5.15)
  line L358 (21.6, -5.15) -> (21.9, -5.15)
  line L359 (21.6, -6.35) -> (21.6, -5.15)
  line L360 (21.9, -6.35) -> (21.6, -6.35)
  line L361 (21.9, -5.15) -> (21.9, -6.35)
  line L362 (21.9, 5.15) -> (21.6, 5.15)
  line L363 (22.1, 6.35) -> (22.4, 6.35)
  line L364 (22.1, 5.15) -> (22.1, 6.35)
  line L365 (22.4, 6.35) -> (22.4, 5.15)
  line L366 (22.1, -5.15) -> (22.4, -5.15)
  line L367 (22.1, -6.35) -> (22.1, -5.15)
  line L368 (22.4, -6.35) -> (22.1, -6.35)
  line L369 (22.4, -5.15) -> (22.4, -6.35)
  line L370 (22.4, 5.15) -> (22.1, 5.15)
  line L371 (22.6, 6.35) -> (22.9, 6.35)
  line L372 (22.6, 5.15) -> (22.6, 6.35)
  line L373 (22.9, 6.35) -> (22.9, 5.15)
  line L374 (22.6, -5.15) -> (22.9, -5.15)
  line L375 (22.6, -6.35) -> (22.6, -5.15)
  line L376 (22.9, -6.35) -> (22.6, -6.35)
  line L377 (22.9, -5.15) -> (22.9, -6.35)
  line L378 (22.9, 5.15) -> (22.6, 5.15)
  line L379 (23.1, 6.35) -> (23.4, 6.35)
  line L380 (23.1, 5.15) -> (23.1, 6.35)
  line L381 (23.4, 6.35) -> (23.4, 5.15)
  line L382 (23.1, -5.15) -> (23.4, -5.15)
  line L383 (23.1, -6.35) -> (23.1, -5.15)
  line L384 (23.4, -6.35) -> (23.1, -6.35)
  line L385 (23.4, -5.15) -> (23.4, -6.35)
  line L386 (23.4, 5.15) -> (23.1, 5.15)
  line L387 (23.6, 6.35) -> (23.9, 6.35)
  line L388 (23.6, 5.15) -> (23.6, 6.35)
  line L389 (23.9, 6.35) -> (23.9, 5.15)
  line L390 (23.6, -5.15) -> (23.9, -5.15)
  line L391 (23.6, -6.35) -> (23.6, -5.15)
  line L392 (23.9, -6.35) -> (23.6, -6.35)
  line L393 (23.9, -5.15) -> (23.9, -6.35)
  line L394 (23.9, 5.15) -> (23.6, 5.15)
  line L395 (25.15, 3.9) -> (26.35, 3.9)
  line L396 (26.35, 3.9) -> (26.35, 3.6)
  line L397 (26.35, 3.6) -> (25.15, 3.6)
  line L398 (25.15, 3.6) -> (25.15, 3.9)
  line L399 (13.65, 3.9) -> (14.85, 3.9)
  line L400 (14.85, 3.9) -> (14.85, 3.6)
  line L401 (14.85, 3.6) -> (13.65, 3.6)
  line L402 (13.65, 3.6) -> (13.65, 3.9)
  line L403 (14.85, 3.4) -> (14.85, 3.1)
  line L404 (14.85, 3.1) -> (13.65, 3.1)
  line L405 (13.65, 3.4) -> (14.85, 3.4)
  line L406 (13.65, 3.1) -> (13.65, 3.4)
  line L407 (25.15, 3.1) -> (25.15, 3.4)
  line L408 (26.35, 3.1) -> (25.15, 3.1)
  line L409 (26.35, 3.4) -> (26.35, 3.1)
  line L410 (25.15, 3.4) -> (26.35, 3.4)
  line L411 (14.85, 2.9) -> (14.85, 2.6)
  line L412 (14.85, 2.6) -> (13.65, 2.6)
  line L413 (13.65, 2.9) -> (14.85, 2.9)
  line L414 (13.65, 2.6) -> (13.65, 2.9)
  line L415 (25.15, 2.6) -> (25.15, 2.9)
  line L416 (26.35, 2.6) -> (25.15, 2.6)
  line L417 (26.35, 2.9) -> (26.35, 2.6)
  line L418 (25.15, 2.9) -> (26.35, 2.9)
  line L419 (14.85, 2.4) -> (14.85, 2.1)
  line L420 (14.85, 2.1) -> (13.65, 2.1)
  line L421 (13.65, 2.4) -> (14.85, 2.4)
  line L422 (13.65, 2.1) -> (13.65, 2.4)
  line L423 (25.15, 2.1) -> (25.15, 2.4)
  line L424 (26.35, 2.1) -> (25.15, 2.1)
  line L425 (26.35, 2.4) -> (26.35, 2.1)
  line L426 (25.15, 2.4) -> (26.35, 2.4)
  line L427 (14.85, 1.9) -> (14.85, 1.6)
  line L428 (14.85, 1.6) -> (13.65, 1.6)
  line L429 (13.65, 1.9) -> (14.85, 1.9)
  line L430 (13.65, 1.6) -> (13.65, 1.9)
  line L431 (25.15, 1.6) -> (25.15, 1.9)
  line L432 (26.35, 1.6) -> (25.15, 1.6)
  line L433 (26.35, 1.9) -> (26.35, 1.6)
  line L434 (25.15, 1.9) -> (26.35, 1.9)
  line L435 (14.85, 1.4) -> (14.85, 1.1)
  line L436 (14.85, 1.1) -> (13.65, 1.1)
  line L437 (13.65, 1.4) -> (14.85, 1.4)
  line L438 (13.65, 1.1) -> (13.65, 1.4)
  line L439 (25.15, 1.1) -> (25.15, 1.4)
  line L440 (26.35, 1.1) -> (25.15, 1.1)
  line L441 (26.35, 1.4) -> (26.35, 1.1)
  line L442 (25.15, 1.4) -> (26.35, 1.4)
  line L443 (14.85, 0.9) -> (14.85, 0.6)
  line L444 (14.85, 0.6) -> (13.65, 0.6)
  line L445 (13.65, 0.9) -> (14.85, 0.9)
  line L446 (13.65, 0.6) -> (13.65, 0.9)
  line L447 (25.15, 0.6) -> (25.15, 0.9)
  line L448 (26.35, 0.6) -> (25.15, 0.6)
  line L449 (26.35, 0.9) -> (26.35, 0.6)
  line L450 (25.15, 0.9) -> (26.35, 0.9)
  line L451 (14.85, 0.4) -> (14.85, 0.1)
  line L452 (14.85, 0.1) -> (13.65, 0.1)
  line L453 (13.65, 0.4) -> (14.85, 0.4)
  line L454 (13.65, 0.1) -> (13.65, 0.4)
  line L455 (25.15, 0.1) -> (25.15, 0.4)
  line L456 (26.35, 0.1) -> (25.15, 0.1)
  line L457 (26.35, 0.4) -> (26.35, 0.1)
  line L458 (25.15, 0.4) -> (26.35, 0.4)
  line L459 (14.85, -0.1) -> (14.85, -0.4)
  line L460 (14.85, -0.4) -> (13.65, -0.4)
  line L461 (13.65, -0.1) -> (14.85, -0.1)
  line L462 (13.65, -0.4) -> (13.65, -0.1)
  line L463 (25.15, -0.4) -> (25.15, -0.1)
  line L464 (26.35, -0.4) -> (25.15, -0.4)
  line L465 (26.35, -0.1) -> (26.35, -0.4)
  line L466 (25.15, -0.1) -> (26.35, -0.1)
  line L467 (14.85, -0.6) -> (14.85, -0.9)
  line L468 (14.85, -0.9) -> (13.65, -0.9)
  line L469 (13.65, -0.6) -> (14.85, -0.6)
  line L470 (13.65, -0.9) -> (13.65, -0.6)
  line L471 (25.15, -0.9) -> (25.15, -0.6)
  line L472 (26.35, -0.9) -> (25.15, -0.9)
  line L473 (26.35, -0.6) -> (26.35, -0.9)
  line L474 (25.15, -0.6) -> (26.35, -0.6)
  line L475 (14.85, -1.1) -> (14.85, -1.4)
  line L476 (14.85, -1.4) -> (13.65, -1.4)
  line L477 (13.65, -1.1) -> (14.85, -1.1)
  line L478 (13.65, -1.4) -> (13.65, -1.1)
  line L479 (25.15, -1.4) -> (25.15, -1.1)
  line L480 (26.35, -1.4) -> (25.15, -1.4)
  line L481 (26.35, -1.1) -> (26.35, -1.4)
  line L482 (25.15, -1.1) -> (26.35, -1.1)
  line L483 (14.85, -1.6) -> (14.85, -1.9)
  line L484 (14.85, -1.9) -> (13.65, -1.9)
  line L485 (13.65, -1.6) -> (14.85, -1.6)
  line L486 (13.65, -1.9) -> (13.65, -1.6)
  line L487 (25.15, -1.9) -> (25.15, -1.6)
  line L488 (26.35, -1.9) -> (25.15, -1.9)
  line L489 (26.35, -1.6) -> (26.35, -1.9)
  line L490 (25.15, -1.6) -> (26.35, -1.6)
  line L491 (14.85, -2.1) -> (14.85, -2.4)
  line L492 (14.85, -2.4) -> (13.65, -2.4)
  line L493 (13.65, -2.1) -> (14.85, -2.1)
  line L494 (13.65, -2.4) -> (13.65, -2.1)
  line L495 (25.15, -2.4) -> (25.15, -2.1)
  line L496 (26.35, -2.4) -> (25.15, -2.4)
  line L497 (26.35, -2.1) -> (26.35, -2.4)
  line L498 (25.15, -2.1) -> (26.35, -2.1)
  line L499 (14.85, -2.6) -> (14.85, -2.9)
  line L500 (14.85, -2.9) -> (13.65, -2.9)
  line L501 (13.65, -2.6) -> (14.85, -2.6)
  line L502 (13.65, -2.9) -> (13.65, -2.6)
  line L503 (25.15, -2.9) -> (25.15, -2.6)
  line L504 (26.35, -2.9) -> (25.15, -2.9)
  line L505 (26.35, -2.6) -> (26.35, -2.9)
  line L506 (25.15, -2.6) -> (26.35, -2.6)
  line L507 (14.85, -3.1) -> (14.85, -3.4)
  line L508 (14.85, -3.4) -> (13.65, -3.4)
  line L509 (13.65, -3.1) -> (14.85, -3.1)
  line L510 (13.65, -3.4) -> (13.65, -3.1)
  line L511 (25.15, -3.4) -> (25.15, -3.1)
  line L512 (26.35, -3.4) -> (25.15, -3.4)
  line L513 (26.35, -3.1) -> (26.35, -3.4)
  line L514 (25.15, -3.1) -> (26.35, -3.1)
  line L515 (14.85, -3.6) -> (14.85, -3.9)
  line L516 (14.85, -3.9) -> (13.65, -3.9)
  line L517 (13.65, -3.6) -> (14.85, -3.6)
  line L518 (13.65, -3.9) -> (13.65, -3.6)
  line L519 (25.15, -3.9) -> (25.15, -3.6)
  line L520 (26.35, -3.9) -> (25.15, -3.9)
  line L521 (26.35, -3.6) -> (26.35, -3.9)
  line L522 (25.15, -3.6) -> (26.35, -3.6)
  line L523 (13.65, 6.35) -> (26.35, 6.35) construction
  line L524 (26.35, 6.35) -> (26.35, -6.35) construction
  line L525 (26.35, -6.35) -> (13.65, -6.35) construction
  line L526 (13.65, -6.35) -> (13.65, 6.35) construction
  line L527 (13.65, 0) -> (26.35, 0) construction
  line L528 (20, 6.35) -> (20, -6.35) construction
  line L529 (12.1, 6.73) -> (13.2, 6.73)
  line L530 (13.2, 6.73) -> (13.2, 5.63)
  line L531 (13.2, 5.63) -> (12.1, 5.63)
  line L532 (12.1, 5.63) -> (12.1, 6.73)
  line L533 (12.1, 5) -> (13.2, 5)
  line L534 (13.2, 5) -> (13.2, 3.9)
  line L535 (13.2, 3.9) -> (12.1, 3.9)
  line L536 (12.1, 3.9) -> (12.1, 5)
  line L537 (15, -6.8) -> (16.1, -6.8)
  line L538 (13.27, -6.8) -> (14.37, -6.8)
  line L539 (16.1, -6.8) -> (16.1, -7.9)
  line L540 (16.1, -7.9) -> (15, -7.9)
  line L541 (15, -7.9) -> (15, -6.8)
  line L542 (14.37, -6.8) -> (14.37, -7.9)
  line L543 (13.27, -7.9) -> (13.27, -6.8)
  line L544 (14.37, -7.9) -> (13.27, -7.9)
  line L545 (26.8, -5) -> (26.8, -3.9)
  line L546 (26.8, -6.73) -> (26.8, -5.63)
  line L547 (26.8, -3.9) -> (27.9, -3.9)
  line L548 (27.9, -3.9) -> (27.9, -5)
  line L549 (27.9, -5) -> (26.8, -5)
  line L550 (26.8, -5.63) -> (27.9, -5.63)
  line L551 (27.9, -6.73) -> (26.8, -6.73)
  line L552 (27.9, -5.63) -> (27.9, -6.73)
  line L553 (25, 6.8) -> (23.9, 6.8)
  line L554 (26.73, 6.8) -> (25.63, 6.8)
  line L555 (23.9, 6.8) -> (23.9, 7.9)
  line L556 (23.9, 7.9) -> (25, 7.9)
  line L557 (25, 7.9) -> (25, 6.8)
  line L558 (25.63, 6.8) -> (25.63, 7.9)
  line L559 (26.73, 7.9) -> (26.73, 6.8)
  line L560 (25.63, 7.9) -> (26.73, 7.9)
  line L561 (14.65, 12.88) -> (15.75, 12.88)
  line L562 (15.75, 12.88) -> (15.75, 11.78)
  line L563 (15.75, 11.78) -> (14.65, 11.78)
  line L564 (14.65, 11.78) -> (14.65, 12.88)
  line L565 (14.65, 11.15) -> (15.75, 11.15)
  line L566 (15.75, 11.15) -> (15.75, 10.05)
  line L567 (15.75, 10.05) -> (14.65, 10.05)
  line L568 (14.65, 10.05) -> (14.65, 11.15)
  line L569 (17.65, 12.88) -> (18.75, 12.88)
  line L570 (18.75, 12.88) -> (18.75, 11.78)
  line L571 (18.75, 11.78) -> (17.65, 11.78)
  line L572 (17.65, 11.78) -> (17.65, 12.88)
  line L573 (17.65, 11.15) -> (18.75, 11.15)
  line L574 (18.75, 11.15) -> (18.75, 10.05)
  line L575 (18.75, 10.05) -> (17.65, 10.05)
  line L576 (17.65, 10.05) -> (17.65, 11.15)
  line L577 (18.9, 9.75) -> (17.5, 9.75)
  line L578 (17.5, 9.75) -> (17.5, 8.6)
  line L579 (17.5, 8.6) -> (18.9, 8.6)
  line L580 (18.9, 8.6) -> (18.9, 9.75)
  line L581 (18.9, 7) -> (17.5, 7)
  line L582 (17.5, 7) -> (17.5, 8.15)
  line L583 (17.5, 8.15) -> (18.9, 8.15)
  line L584 (18.9, 8.15) -> (18.9, 7)
  line L585 (15.9, 7) -> (14.5, 7)
  line L586 (14.5, 7) -> (14.5, 8.15)
  line L587 (14.5, 8.15) -> (15.9, 8.15)
  line L588 (15.9, 8.15) -> (15.9, 7)
  line L589 (14.5, 8.6) -> (15.9, 8.6)
  line L590 (15.9, 8.6) -> (15.9, 9.75)
  line L591 (15.9, 9.75) -> (14.5, 9.75)
  line L592 (14.5, 9.75) -> (14.5, 8.6)
  line L593 (23.4831, 10.3536) -> (22.3831, 10.3536)
  line L594 (25.2131, 10.3536) -> (24.1131, 10.3536)
  line L595 (22.3831, 10.3536) -> (22.3831, 11.4536)
  line L596 (22.3831, 11.4536) -> (23.4831, 11.4536)
  line L597 (23.4831, 11.4536) -> (23.4831, 10.3536)
  line L598 (24.1131, 10.3536) -> (24.1131, 11.4536)
  line L599 (25.2131, 11.4536) -> (25.2131, 10.3536)
  line L600 (24.1131, 11.4536) -> (25.2131, 11.4536)
  point P0 (0, 0)
  point P1 (12.65, 5.63)
  point P2 (12.65, 5)
  point P3 (12.1, 6.18)
  point P4 (12.1, 4.45)
  point P5 (20, 0)
  point P6 (14.37, -7.35)
  point P7 (15, -7.35)
  point P8 (15.55, -7.9)
  point P9 (13.82, -7.9)
  point P10 (27.35, -5.63)
  point P11 (27.35, -5)
  point P12 (27.9, -4.45)
  point P13 (27.9, -6.18)
  point P14 (25.63, 7.35)
  point P15 (25, 7.35)
  point P16 (24.45, 7.9)
  point P17 (26.18, 7.9)
  point P18 (15.2, 11.78)
  point P19 (15.2, 11.15)
  point P20 (14.65, 12.33)
  point P21 (14.65, 10.6)
  point P22 (18.2, 11.78)
  point P23 (18.2, 11.15)
  point P24 (17.65, 12.33)
  point P25 (17.65, 10.6)
  point P26 (18.2, 9.75)
  point P27 (18.2, 10.05)
  point P28 (22.9331, 11.4536)
  point P29 (24.6631, 11.4536)
  dimension "d68" = 1
  dimension "d69" = 2.5
  dimension "d72" = 2.54
  dimension "d77" = 18
  dimension "d78" = 25
  dimension "d79" = 10.3
  dimension "d80" = 12.7
  dimension "d81" = 0.3
  dimension "d84" = 0.5
  dimension "d91" = 0.5
  dimension "d96" = 3.9
  dimension "d97" = 20
  dimension "d98" = 3.9
  dimension "d123" = 1.1
  dimension "d124" = 1.1
  dimension "d125" = 1.73
  dimension "d126" = 1
  dimension "d127" = 5
  dimension "d130" = 360
  dimension "d148" = 1.73
  dimension "d166" = 3
  dimension "d167" = 1.4
  dimension "d168" = 1.6
  dimension "d169" = 1.15
  dimension "d170" = 0.45
  dimension "d171" = 1.8
  dimension "d172" = 7
  dimension "d173" = 0.3
  dimension "d189" = 2.3831
  dimension "d190" = 10.3536
  dimension "d191" = 1.73
  constraints: 716 end point, 54 point on line, 32 parallel, 21 midpoint, 18 equal length, 18 horizontal, 18 perpendicular, 12 collinear, 4 vertical alignment, 1 vertical, 601 other
  measures "d68" distance of L243.start L243.end
  measures "d69" distance of L245.end L243.start
  measures "d72" distance of L244.end L247.start
  measures "d77" distance from line of L246 point (0, 0)
  measures "d78" distance from line of L243 point (0, 0)
  measures "d79" distance between parallel lines of L271 L269
  measures "d80" distance between parallel lines of L273 L267
  measures "d81" distance of L267.start L267.end
  measures "d84" distance of L267.start L275.start
  measures "d91" distance of L400.end L403.end
  measures "d96" distance between parallel lines of L399 L527
  measures "d97" distance between parallel lines of L528 L234
  measures "d98" distance between parallel lines of L528 L270
  measures "d123" distance of L529.start L529.end
  measures "d124" distance of L531.end L529.start
  measures "d125" distance of point (12.1, 4.45) point (12.1, 6.18)
  measures "d126" distance from line of L526 point (12.65, 5)
  measures "d127" distance between parallel lines of L533 L527
  measures "d148" distance of point (14.65, 10.6) point (14.65, 12.33)
  measures "d166" distance of point (15.2, 11.78) point (18.2, 11.78)
  measures "d167" distance of L581.start L581.end
  measures "d168" distance between parallel lines of L588 L582
  measures "d169" distance of L585.end L586.end
  measures "d170" distance between parallel lines of L589 L587
  measures "d171" distance from line of point (18.2, 9.75) L528
  measures "d172" distance between parallel lines of L581 L527
  measures "d173" distance between parallel lines of L575 L577
  measures "d189" distance between parallel lines of L528 L595
  measures "d190" distance between parallel lines of L527 L593
  measures "d191" distance of point (22.933, 11.454) point (24.663, 11.454)
extrude "Extrusion6" add sketch "Sketch6" along normal blind 0.035 contours L243 L244 L245 L246 | L247 L250 L249 L248 | L251 L254 L253 L252 | L255 L258 L257 L256 | L259 L262 L261 L260 | L263 L266 L265 L264 | L267 L268 L269 L270 | L271 L272 L273 L274 | L275 L277 L282 L276 | L278 L281 L280 L279 | L283 L285 L290 L284 | L286 L289 L288 L287 | L291 L293 L298 L292 | L294 L297 L296 L295 | L299 L301 L306 L300 | L302 L305 L304 L303 | L307 L309 L314 L308 | L310 L313 L312 L311 | L315 L317 L322 L316 | L318 L321 L320 L319 | L323 L325 L330 L324 | L326 L329 L328 L327 | L331 L333 L338 L332 | L334 L337 L336 L335 | L339 L341 L346 L340 | L342 L345 L344 L343 | L347 L349 L354 L348 | L350 L353 L352 L351 | L355 L357 L362 L356 | L358 L361 L360 L359 | L363 L365 L370 L364 | L366 L369 L368 L367 | L371 L373 L378 L372 | L374 L377 L376 L375 | L379 L381 L386 L380 | L382 L385 L384 L383 | L387 L389 L394 L388 | L390 L393 L392 L391 | L395 L396 L397 L398 | L399 L400 L401 L402 | L403 L404 L406 L405 | L407 L410 L409 L408 | L411 L412 L414 L413 | L415 L418 L417 L416 | L419 L420 L422 L421 | L423 L426 L425 L424 | L427 L428 L430 L429 | L431 L434 L433 L432 | L435 L436 L438 L437 | L439 L442 L441 L440 | L443 L444 L446 L445 | L447 L450 L449 L448 | L451 L452 L454 L453 | L455 L458 L457 L456 | L459 L460 L462 L461 | L463 L466 L465 L464 | L467 L468 L470 L469 | L471 L474 L473 L472 | L475 L476 L478 L477 | L479 L482 L481 L480 | L483 L484 L486 L485 | L487 L490 L489 L488 | L491 L492 L494 L493 | L495 L498 L497 L496 | L499 L500 L502 L501 | L503 L506 L505 L504 | L507 L508 L510 L509 | L511 L514 L513 L512 | L515 L516 L518 L517 | L519 L522 L521 L520 | L529 L530 L531 L532 | L533 L534 L535 L536 | L537 L539 L540 L541 | L538 L542 L544 L543 | L545 L547 L548 L549 | L546 L550 L552 L551 | L553 L555 L556 L557 | L554 L558 L560 L559 | L561 L562 L563 L564 | L565 L566 L567 L568 | L569 L570 L571 L572 | L573 L574 L575 L576 | L580 L579 L578 L577 | L581 L582 L583 L584 | L585 L586 L587 L588 | L592 L591 L590 L589 | L593 L595 L596 L597 | L594 L598 L600 L599